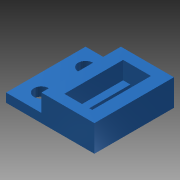
# Autodesk Inventor part: switch lever 2
Saved by Autodesk Inventor 2013 (Build 170138000, 138)
## iProperties
Created: 2017-02-23
Part Number: switch lever 2
Material: Generic
Document SubType Name: Modeling
Designer: Herman de Vries
Density: 1 g/cm^3
Author: Herman de Vries
Autodesk Inventor part; units mm, degrees
ref_plane "YZ Plane" through (0, 0, 0) normal (1, 0, 0) x (0, 1, 0)
ref_plane "XZ Plane" through (0, 0, 0) normal (0, 1, 0) x (-1, 0, 0)
ref_plane "XY Plane" through (0, 0, 0) normal (0, 0, 1) x (1, 0, 0)
sketch "Sketch1" plane through (0, 0, 0) normal (0, 0, 1) x (1, 0, 0)
  line L0 (0, 0) -> (20, 0)
  line L1 (20, 0) -> (20, 18)
  line L2 (20, 18) -> (0, 18)
  line L3 (0, 18) -> (0, 0)
  line L4 (12.5, 2.35) -> (15.5, 2.35)
  line L5 (15.5, 2.35) -> (15.5, 15.65)
  line L6 (15.5, 15.65) -> (12.5, 15.65)
  line L7 (12.5, 15.65) -> (12.5, 2.35)
  circle A0 centre (4, 14) radius 1.7
  circle A1 centre (4, 4) radius 1.7
  line L8 (20, 18) -> (8, 18)
  line L9 (8, 18) -> (8, 0)
  line L10 (8, 0) -> (20, 0)
  line L11 (20, 0) -> (20, 18)
  line L12 (10.85, 15.65) -> (17.15, 15.65)
  line L13 (17.15, 15.65) -> (17.15, 2.35)
  line L14 (17.15, 2.35) -> (10.85, 2.35)
  line L15 (10.85, 2.35) -> (10.85, 15.65)
  point P0 (15.5, 9)
  point P1 (20, 9)
  point P2 (14, 15.65)
  point P3 (14, 18)
  point P4 (17.15, 9)
  point P5 (20, 9)
  point P6 (14, 15.65)
  dimension "d0" = 20
  dimension "d1" = 18
  dimension "d3" = 3
  dimension "d5" = 3.4
  dimension "d6" = 3.4
  dimension "d7" = 4
  dimension "d8" = 4
  dimension "d9" = 10
  dimension "d20" = 12
  dimension "d21" = 6.3
  dimension "d22" = 13.3
  constraints: 32 end point, 8 parallel, 7 midpoint, 4 horizontal, 4 perpendicular, 2 centre point, 2 horizontal alignment, 2 vertical alignment, 1 coincident, 1 collinear, 1 point on line
  measures "d0" distance of L0.start L0.end
  measures "d1" distance of L0.end L1.end
  measures "d3" distance of L4.start L4.end
  measures "d5" diameter of A0
  measures "d6" diameter of A1
  measures "d7" distance from line of L3 A0.centre
  measures "d8" distance from line of L0 A1.centre
  measures "d9" distance of A0.centre A1.centre
  measures "d20" distance of L10.end L9.end
  measures "d21" distance of L12.start L12.end
  measures "d22" distance of L14.end L12.start
extrude "Extrusion1" add sketch "Sketch1" along normal blind 2 contours L3 L2 L9 L0 | L9 L2 L1 L0 | L14 L15 L12 L7 | L5 L12 L13 L14
extrude "Extrusion3" add sketch "Sketch1" along normal blind 6 contours L9 L2 L1 L0
body "Solid1"
